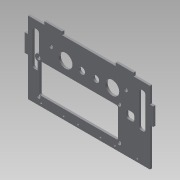
# Autodesk Inventor part: Kepala Tutup belakang
Saved by Autodesk Inventor 2015 SP1 (Build 190203100, 203)
## iProperties
Created: 2015-04-11
Part Number: Kepala Tutup belakang
Material: Generic
Document SubType Name: Modeling
Designer: Rafi Kurnia Putra
Density: 1 g/cm^3
Appearance: Default
Author: Rafi Kurnia Putra
Autodesk Inventor part; units mm, degrees
(part 1 of 2)
ref_plane "YZ Plane" through (0, 0, 0) normal (1, 0, 0) x (0, 1, 0)
ref_plane "XZ Plane" through (0, 0, 0) normal (0, 1, 0) x (-1, 0, 0)
ref_plane "XY Plane" through (0, 0, 0) normal (0, 0, 1) x (1, 0, 0)
sketch "Sketch1" plane through (0, 0, 0) normal (0, 1, 0) x (-1, 0, 0)
  circle A0 centre (-10.5001, 30.1708) radius 1
  circle A1 centre (10.4999, 30.1712) radius 1
  circle A2 centre (23.9063, 30.1714) radius 1
  circle A3 centre (-44.9057, 30.1702) radius 1
  circle A4 centre (44.9063, 30.1718) radius 1
  circle A5 centre (-23.9057, 30.1706) radius 1
  circle A6 centre (47.0718, 65.4919) radius 1.75
  circle A7 centre (47.0718, 34.2919) radius 1.75
  circle A8 centre (-28.1782, 34.2919) radius 1.75
  circle A9 centre (-28.1782, 65.4919) radius 1.75
  circle A10 centre (-6.604, 75.238) radius 3
  circle A11 centre (6.604, 75.238) radius 3
  circle A12 centre (-34.465, 80.373) radius 1.75
  circle A13 centre (35.535, 80.373) radius 1.75
  circle A14 centre (-21.844, 75.746) radius 6.43
  circle A15 centre (21.844, 75.746) radius 6.43
  line L0 (58.58, 79.6254) -> (58.58, 122) construction
  line L1 (-57.0002, 27.1688) -> (-57.0005, 63.0729)
  line L2 (-57.0005, 63.0729) -> (-60.0005, 63.0729)
  line L3 (-60.0005, 63.0729) -> (-60.0005, 79.762)
  line L4 (-60.0005, 79.762) -> (-57.0005, 79.762)
  line L5 (-57.0005, 79.762) -> (-57.0005, 94.8331)
  line L6 (-57.0005, 94.8331) -> (-41.6794, 94.8331)
  line L7 (-41.6794, 94.8331) -> (-41.6794, 97.8331)
  line L8 (-41.6794, 97.8331) -> (-24.9903, 97.8331)
  line L9 (-24.9903, 97.8331) -> (-24.9903, 94.8331)
  line L10 (-24.9903, 94.8331) -> (24.9903, 94.8331)
  line L11 (24.9903, 94.8331) -> (24.9903, 97.8331)
  line L12 (24.9903, 97.8331) -> (41.6794, 97.8331)
  line L13 (41.6794, 97.8331) -> (41.6794, 94.8331)
  line L14 (41.6794, 94.8331) -> (57.0005, 94.8331)
  line L15 (57.0005, 94.8331) -> (57.0005, 79.762)
  line L16 (57.0005, 79.762) -> (59.9995, 79.762)
  line L17 (59.9995, 79.762) -> (59.9998, 63.0742)
  line L18 (59.9998, 63.0742) -> (56.9998, 63.0741)
  line L19 (56.9998, 63.0741) -> (57.0002, 27.1688)
  line L20 (45.2968, 36.8919) -> (-26.4032, 36.8919)
  line L21 (-26.4032, 36.8919) -> (-26.4032, 62.8919)
  line L22 (-26.4032, 62.8919) -> (45.2968, 62.8919)
  line L23 (45.2968, 62.8919) -> (45.2968, 36.8919)
  line L24 (-46.6476, 56.7523) -> (-46.6476, 85.7402)
  line L25 (-48.6476, 87.7402) -> (-50.6476, 87.7402)
  line L26 (-52.6476, 85.7402) -> (-52.6476, 56.7523)
  line L27 (-50.6476, 54.7523) -> (-48.6476, 54.7523)
  arc A16 (-46.6476, 85.7402) -> (-48.6476, 87.7402) centre (-48.6476, 85.7402) ccw
  arc A17 (-50.6476, 87.7402) -> (-52.6476, 85.7402) centre (-50.6476, 85.7402) ccw
  arc A18 (-52.6476, 56.7523) -> (-50.6476, 54.7523) centre (-50.6476, 56.7523) ccw
  arc A19 (-48.6476, 54.7523) -> (-46.6476, 56.7523) centre (-48.6476, 56.7523) ccw
  line L28 (-48.6476, 56.7523) -> (-50.6476, 85.7402) construction
  line L29 (-50.6476, 56.7523) -> (-48.6476, 85.7402) construction
  line L30 (0.035, 14) -> (0.035, 26) construction
  arc A20 (50.7176, 54.7523) -> (52.7176, 56.7523) centre (50.7176, 56.7523) ccw
  arc A21 (46.7176, 56.7523) -> (48.7176, 54.7523) centre (48.7176, 56.7523) ccw
  line L31 (50.7176, 54.7523) -> (48.7176, 54.7523)
  line L32 (52.7176, 85.7402) -> (52.7176, 56.7523)
  arc A22 (48.7176, 87.7402) -> (46.7176, 85.7402) centre (48.7176, 85.7402) ccw
  line L33 (48.7176, 87.7402) -> (50.7176, 87.7402)
  arc A23 (52.7176, 85.7402) -> (50.7176, 87.7402) centre (50.7176, 85.7402) ccw
  line L34 (48.7176, 56.7523) -> (50.7176, 85.7402) construction
  line L35 (50.7176, 56.7523) -> (48.7176, 85.7402) construction
  arc A24 (46.7176, 62.1619) -> (46.7176, 68.822) centre (47.0718, 65.4919) ccw
  line L36 (46.7176, 56.7523) -> (46.7176, 62.1619)
  line L37 (46.7176, 63.7782) -> (46.7176, 62.8919)
  line L38 (46.7176, 68.822) -> (46.7176, 85.7402)
  line L39 (57.0002, 27.1688) -> (-57.0002, 27.1688)
  line L40 (-36.8282, 57.7419) -> (-40.3282, 57.7419)
  line L41 (-42.3282, 59.7419) -> (-42.3282, 63.2419)
  line L42 (-40.3282, 65.2419) -> (-36.8282, 65.2419)
  line L43 (-34.8282, 63.2419) -> (-34.8282, 59.7419)
  line L44 (-34.8282, 57.7419) -> (-42.3282, 65.2419) construction
  line L45 (-42.3282, 57.7419) -> (-34.8282, 65.2419) construction
  arc A25 (-36.8282, 57.7419) -> (-34.8282, 59.7419) centre (-36.8282, 59.7419) ccw
  arc A26 (-42.3282, 59.7419) -> (-40.3282, 57.7419) centre (-40.3282, 59.7419) ccw
  arc A27 (-40.3282, 65.2419) -> (-42.3282, 63.2419) centre (-40.3282, 63.2419) ccw
  arc A28 (-34.8282, 63.2419) -> (-36.8282, 65.2419) centre (-36.8282, 63.2419) ccw
  line L46 (-27.2951, 36) -> (46.1888, 36)
  line L47 (46.1888, 36) -> (46.1888, 63.7839)
  line L48 (46.1888, 63.7839) -> (-27.2951, 63.7839)
  line L49 (-27.2951, 63.7839) -> (-27.2951, 36)
  point P0 (-49.6476, 71.2463)
  point P1 (-60.0005, 71.2463)
  point P2 (49.7176, 71.2463)
  point P3 (0, 73.6476)
  point P4 (-28.274, 68.5919)
  point P5 (35.535, 92.123)
  point P6 (-38.5782, 61.4919)
  dimension "d20" = 6
  dimension "d21" = 0
  dimension "d22" = 7.353
  dimension "d23" = 1.5989
  dimension "d27" = 43.688
  dimension "d28" = 21.844
  dimension "d30" = 3.1
  dimension "d32" = 11.75
  dimension "d33" = 6
  dimension "d34" = 6.604
  dimension "d35" = 6.604
  dimension "d38" = 13.691
  dimension "d45" = 70
  dimension "d52" = 7.5
  dimension "d53" = 2
  dimension "d61" = 26
  dimension "d62" = 71.7
  dimension "d63" = 31.2
  dimension "d64" = 75.25
  dimension "d67" = 2.6
  dimension "d70" = 1.775
  dimension "d71" = 10.4
  dimension "d74" = 0.8919
  constraints: 100 end point, 28 centre point, 26 point on circle, 16 tangent, 13 symmetric about line, 10 point on line, 9 parallel, 4 midpoint, 4 perpendicular, 3 equal radius, 3 horizontal, 2 horizontal alignment, 2 vertical, 2 vertical alignment, 12 other
  measures "d20" distance between parallel lines of L26 L24
  measures "d21" vertical distance of point (-49.648, 71.246) point (-60.001, 71.246)
  measures "d22" distance from line of L1 point (-49.648, 71.246)
  measures "d27" distance of A14.centre A15.centre
  measures "d28" horizontal distance of point (0, 73.648) A15.centre
  measures "d30" vertical distance of point (-28.274, 68.592) A9.centre
  measures "d32" distance of point (35.535, 92.123) A13.centre
  measures "d33" diameter of A10
  measures "d34" horizontal distance of A10.centre point (0, 73.648)
  measures "d35" horizontal distance of A11.centre point (0, 73.648)
  measures "d38" horizontal distance of A15.centre A13.centre
  measures "d45" distance of A12.centre A13.centre
  measures "d52" distance of L45.start L44.end
  measures "d53" radius of A25
  measures "d61" distance between parallel lines of L22 L20
  measures "d62" distance between parallel lines of L21 L23
  measures "d63" distance of A9.centre A8.centre
  measures "d64" distance of A8.centre A7.centre
  measures "d67" distance from line of A7.centre L20
  measures "d70" distance from line of A7.centre L23
  measures "d71" horizontal distance of point (-38.578, 61.492) A9.centre
  measures "d74" distance between parallel lines of L20 L46
extrude "Extrusion1" add sketch "Sketch1" along normal blind 2 contours L1 L2 L3 L4 L5 L6 L7 L8 L9 L10 L11 L12 L13 L14 L15 L16 L17 L18 L19 L39 | L40 A26 L41 A27 L42 A28 L43 A25 | L49 L48 L47 L46
sketch "Sketch2" plane through (0, 2, 0) normal (0, 1, 0) x (1, 0, 0)
  line L0 (-22.4709, -80.6452) -> (21.8526, -80.6452) construction
  line L1 (21.8526, -80.6452) -> (21.8526, -96.7887) construction
  line L2 (21.8526, -96.7887) -> (-22.4709, -96.7887) construction
  line L3 (-22.4709, -96.7887) -> (-22.4709, -80.6452) construction
  line L4 (38.4446, -27.4209) -> (45.2182, -27.4209) construction
  line L5 (45.2182, -27.4209) -> (45.2182, -65.4969) construction
  line L6 (45.2182, -65.4969) -> (38.4446, -65.4969) construction
  line L7 (38.4446, -65.4969) -> (38.4446, -27.4209) construction
  spline S0 degree 2 poles (-35.3902, -91.377) (-36.3991, -91.377) (-37.485, -90.4046) (-37.485, -89.4645) knots 0 0 0 1 2 2 2
  line L8 (-37.485, -89.4645) -> (-37.485, -86.2717)
  line L9 (-37.485, -86.2717) -> (-36.2289, -86.2717)
  line L10 (-36.2289, -86.2717) -> (-36.2289, -89.3916)
  spline S1 degree 2 poles (-36.2289, -89.3916) (-36.2289, -89.9143) (-35.8359, -90.4248) (-35.3902, -90.4248) knots 0 0 0 1 2 2 2
  spline S2 degree 2 poles (-35.3902, -90.4248) (-34.9566, -90.4248) (-34.5514, -89.9346) (-34.5514, -89.3916) knots 0 0 0 1 2 2 2
  line L11 (-34.5514, -89.3916) -> (-34.5514, -86.2717)
  line L12 (-34.5514, -86.2717) -> (-33.2953, -86.2717)
  line L13 (-33.2953, -86.2717) -> (-33.2953, -89.4605)
  spline S3 degree 2 poles (-33.2953, -89.4605) (-33.2953, -90.3843) (-34.3529, -91.377) (-35.3902, -91.377) knots 0 0 0 1 2 2 2
  line L14 (-28.8707, -91.2717) -> (-30.0539, -91.2717)
  line L15 (-30.0539, -91.2717) -> (-30.0539, -89.4038)
  spline S4 degree 2 poles (-30.0539, -89.4038) (-30.0539, -89.1728) (-30.0903, -88.719) (-30.1389, -88.6137) knots 0 0 0 1 2 2 2
  spline S5 degree 2 poles (-30.1389, -88.6137) (-30.1997, -88.484) (-30.4266, -88.3746) (-30.6211, -88.3746) knots 0 0 0 1 2 2 2
  spline S6 degree 2 poles (-30.6211, -88.3746) (-30.7629, -88.3746) (-31.0587, -88.484) (-31.2248, -88.6015) knots 0 0 0 1 2 2 2
  line L16 (-31.2248, -88.6015) -> (-31.2248, -91.2717)
  line L17 (-31.2248, -91.2717) -> (-32.3999, -91.2717)
  line L18 (-32.3999, -91.2717) -> (-32.3999, -87.4994)
  line L19 (-32.3999, -87.4994) -> (-31.2248, -87.4994)
  line L20 (-31.2248, -87.4994) -> (-31.2248, -87.9167)
  spline S7 degree 2 poles (-31.2248, -87.9167) (-30.9372, -87.6736) (-30.3902, -87.3981) (-30.0579, -87.3981) knots 0 0 0 1 2 2 2
  spline S8 degree 2 poles (-30.0579, -87.3981) (-29.4825, -87.3981) (-28.8707, -88.1274) (-28.8707, -88.8162) knots 0 0 0 1 2 2 2
  line L21 (-28.8707, -88.8162) -> (-28.8707, -91.2717)
  line L22 (-26.8245, -91.2717) -> (-27.9996, -91.2717)
  line L23 (-27.9996, -91.2717) -> (-27.9996, -87.4994)
  line L24 (-27.9996, -87.4994) -> (-26.8245, -87.4994)
  line L25 (-26.8245, -87.4994) -> (-26.8245, -91.2717)
  line L26 (-26.788, -86.9605) -> (-28.032, -86.9605)
  line L27 (-28.032, -86.9605) -> (-28.032, -86.0448)
  line L28 (-28.032, -86.0448) -> (-26.788, -86.0448)
  line L29 (-26.788, -86.0448) -> (-26.788, -86.9605)
  line L30 (-22.3958, -87.4994) -> (-23.7492, -91.2717)
  line L31 (-23.7492, -91.2717) -> (-25.0336, -91.2717)
  line L32 (-25.0336, -91.2717) -> (-26.3748, -87.4994)
  line L33 (-26.3748, -87.4994) -> (-25.1389, -87.4994)
  line L34 (-25.1389, -87.4994) -> (-24.3691, -89.9913)
  line L35 (-24.3691, -89.9913) -> (-23.6073, -87.4994)
  line L36 (-23.6073, -87.4994) -> (-22.3958, -87.4994)
  spline S9 degree 2 poles (-20.0133, -91.373) (-21.083, -91.373) (-22.2216, -90.3519) (-22.2216, -89.4078) knots 0 0 0 1 2 2 2
  spline S10 degree 2 poles (-22.2216, -89.4078) (-22.2216, -88.484) (-21.16, -87.3819) (-20.2038, -87.3819) knots 0 0 0 1 2 2 2
  spline S11 degree 2 poles (-20.2038, -87.3819) (-19.3407, -87.3819) (-18.4655, -88.3179) (-18.4655, -89.185) knots 0 0 0 1 2 2 2
  line L37 (-18.4655, -89.185) -> (-18.4655, -89.6104)
  line L38 (-18.4655, -89.6104) -> (-21.0466, -89.6104)
  spline S12 degree 2 poles (-21.0466, -89.6104) (-21.0303, -89.8738) (-20.8399, -90.2222) (-20.6859, -90.3276) knots 0 0 0 1 2 2 2
  spline S13 degree 2 poles (-20.6859, -90.3276) (-20.536, -90.4329) (-20.1308, -90.5221) (-19.8918, -90.5221) knots 0 0 0 1 2 2 2
  spline S14 degree 2 poles (-19.8918, -90.5221) (-19.6892, -90.5221) (-19.2921, -90.4329) (-19.126, -90.356) knots 0 0 0 1 2 2 2
  spline S15 degree 2 poles (-19.126, -90.356) (-18.9801, -90.2952) (-18.737, -90.1453) (-18.66, -90.0885) knots 0 0 0 1 2 2 2
  line L39 (-18.66, -90.0885) -> (-18.5344, -90.0885)
  line L40 (-18.5344, -90.0885) -> (-18.5344, -91.061)
  spline S16 degree 2 poles (-18.5344, -91.061) (-18.6803, -91.1177) (-18.9153, -91.215) (-19.126, -91.2636) knots 0 0 0 1 2 2 2
  spline S17 degree 2 poles (-19.126, -91.2636) (-19.3164, -91.3162) (-19.7216, -91.373) (-20.0133, -91.373) knots 0 0 0 1 2 2 2
  spline S18 degree 2 poles (-19.6244, -88.9013) (-19.6325, -88.5286) (-19.9607, -88.1355) (-20.297, -88.1355) knots 0 0 0 1 2 2 2
  spline S19 degree 2 poles (-20.297, -88.1355) (-20.6414, -88.1355) (-21.0303, -88.5488) (-21.0506, -88.9013) knots 0 0 0 1 2 2 2
  line L41 (-21.0506, -88.9013) -> (-19.6244, -88.9013)
  line L42 (-15.3294, -88.6137) -> (-15.4266, -88.6137)
  spline S20 degree 2 poles (-15.4266, -88.6137) (-15.4955, -88.5893) (-15.7508, -88.565) (-15.9047, -88.565) knots 0 0 0 1 2 2 2
  spline S21 degree 2 poles (-15.9047, -88.565) (-16.0871, -88.565) (-16.4963, -88.6744) (-16.6868, -88.7474) knots 0 0 0 1 2 2 2
  line L43 (-16.6868, -88.7474) -> (-16.6868, -91.2717)
  line L44 (-16.6868, -91.2717) -> (-17.8618, -91.2717)
  line L45 (-17.8618, -91.2717) -> (-17.8618, -87.4994)
  line L46 (-17.8618, -87.4994) -> (-16.6868, -87.4994)
  line L47 (-16.6868, -87.4994) -> (-16.6868, -88.0423)
  spline S22 degree 2 poles (-16.6868, -88.0423) (-16.6057, -87.9694) (-16.3221, -87.7425) (-16.2046, -87.6736) knots 0 0 0 1 2 2 2
  spline S23 degree 2 poles (-16.2046, -87.6736) (-16.0749, -87.5966) (-15.7346, -87.4872) (-15.5846, -87.4872) knots 0 0 0 1 2 2 2
  spline S24 degree 2 poles (-15.5846, -87.4872) (-15.5279, -87.4872) (-15.3861, -87.4953) (-15.3294, -87.4994) knots 0 0 0 1 2 2 2
  line L48 (-15.3294, -87.4994) -> (-15.3294, -88.6137)
  spline S25 degree 2 poles (-13.7329, -91.373) (-14.1462, -91.373) (-14.8877, -91.1906) (-15.1308, -91.0691) knots 0 0 0 1 2 2 2
  line L49 (-15.1308, -91.0691) -> (-15.1308, -90.0764)
  line L50 (-15.1308, -90.0764) -> (-15.0336, -90.0764)
  spline S26 degree 2 poles (-15.0336, -90.0764) (-14.9485, -90.1412) (-14.7338, -90.2952) (-14.5433, -90.3803) knots 0 0 0 1 2 2 2
  spline S27 degree 2 poles (-14.5433, -90.3803) (-14.3772, -90.4573) (-13.968, -90.5667) (-13.7248, -90.5667) knots 0 0 0 1 2 2 2
  spline S28 degree 2 poles (-13.7248, -90.5667) (-13.4777, -90.5667) (-13.0968, -90.4127) (-13.0968, -90.2466) knots 0 0 0 1 2 2 2
  spline S29 degree 2 poles (-13.0968, -90.2466) (-13.0968, -90.1169) (-13.271, -89.9791) (-13.5222, -89.9224) knots 0 0 0 1 2 2 2
  spline S30 degree 2 poles (-13.5222, -89.9224) (-13.656, -89.8859) (-14.0652, -89.809) (-14.2232, -89.7603) knots 0 0 0 1 2 2 2
  spline S31 degree 2 poles (-14.2232, -89.7603) (-14.6689, -89.6226) (-15.1146, -89.0837) (-15.1146, -88.642) knots 0 0 0 1 2 2 2
  spline S32 degree 2 poles (-15.1146, -88.642) (-15.1146, -88.3908) (-14.8837, -87.9451) (-14.6568, -87.7709) knots 0 0 0 1 2 2 2
  spline S33 degree 2 poles (-14.6568, -87.7709) (-14.4339, -87.6007) (-13.7735, -87.3981) (-13.3561, -87.3981) knots 0 0 0 1 2 2 2
  spline S34 degree 2 poles (-13.3561, -87.3981) (-12.959, -87.3981) (-12.2945, -87.5561) (-12.0676, -87.6655) knots 0 0 0 1 2 2 2
  line L51 (-12.0676, -87.6655) -> (-12.0676, -88.6218)
  line L52 (-12.0676, -88.6218) -> (-12.1608, -88.6218)
  spline S35 degree 2 poles (-12.1608, -88.6218) (-12.2216, -88.5731) (-12.485, -88.4151) (-12.6065, -88.3584) knots 0 0 0 1 2 2 2
  spline S36 degree 2 poles (-12.6065, -88.3584) (-12.7564, -88.2936) (-13.1211, -88.2044) (-13.3115, -88.2044) knots 0 0 0 1 2 2 2
  spline S37 degree 2 poles (-13.3115, -88.2044) (-13.5668, -88.2044) (-13.9193, -88.3786) (-13.9193, -88.5205) knots 0 0 0 1 2 2 2
  spline S38 degree 2 poles (-13.9193, -88.5205) (-13.9193, -88.6501) (-13.7451, -88.796) (-13.4534, -88.8689) knots 0 0 0 1 2 2 2
  spline S39 degree 2 poles (-13.4534, -88.8689) (-13.3034, -88.9054) (-12.9104, -88.9743) (-12.7281, -89.035) knots 0 0 0 1 2 2 2
  spline S40 degree 2 poles (-12.7281, -89.035) (-12.3229, -89.1647) (-11.9015, -89.6712) (-11.9015, -90.0926) knots 0 0 0 1 2 2 2
  spline S41 degree 2 poles (-11.9015, -90.0926) (-11.9015, -90.356) (-12.1487, -90.8381) (-12.3796, -91.0002) knots 0 0 0 1 2 2 2
  spline S42 degree 2 poles (-12.3796, -91.0002) (-12.6187, -91.1785) (-13.2751, -91.373) (-13.7329, -91.373) knots 0 0 0 1 2 2 2
  line L53 (-10.1673, -91.2717) -> (-11.3423, -91.2717)
  line L54 (-11.3423, -91.2717) -> (-11.3423, -87.4994)
  line L55 (-11.3423, -87.4994) -> (-10.1673, -87.4994)
  line L56 (-10.1673, -87.4994) -> (-10.1673, -91.2717)
  line L57 (-10.1308, -86.9605) -> (-11.3748, -86.9605)
  line L58 (-11.3748, -86.9605) -> (-11.3748, -86.0448)
  line L59 (-11.3748, -86.0448) -> (-10.1308, -86.0448)
  line L60 (-10.1308, -86.0448) -> (-10.1308, -86.9605)
  spline S43 degree 2 poles (-7.8253, -91.3446) (-8.5425, -91.3446) (-9.1989, -90.753) (-9.1989, -90.0804) knots 0 0 0 1 2 2 2
  line L61 (-9.1989, -90.0804) -> (-9.1989, -88.3179)
  line L62 (-9.1989, -88.3179) -> (-9.6487, -88.3179)
  line L63 (-9.6487, -88.3179) -> (-9.6487, -87.4994)
  line L64 (-9.6487, -87.4994) -> (-9.1989, -87.4994)
  line L65 (-9.1989, -87.4994) -> (-9.1989, -86.4216)
  line L66 (-9.1989, -86.4216) -> (-8.0239, -86.4216)
  line L67 (-8.0239, -86.4216) -> (-8.0239, -87.4994)
  line L68 (-8.0239, -87.4994) -> (-6.8893, -87.4994)
  line L69 (-6.8893, -87.4994) -> (-6.8893, -88.3179)
  line L70 (-6.8893, -88.3179) -> (-8.0239, -88.3179)
  line L71 (-8.0239, -88.3179) -> (-8.0239, -89.659)
  spline S44 degree 2 poles (-8.0239, -89.659) (-8.0239, -89.8576) (-8.0158, -90.1534) (-7.9671, -90.2709) knots 0 0 0 1 2 2 2
  spline S45 degree 2 poles (-7.9671, -90.2709) (-7.9185, -90.3884) (-7.6795, -90.5261) (-7.4526, -90.5261) knots 0 0 0 1 2 2 2
  spline S46 degree 2 poles (-7.4526, -90.5261) (-7.3553, -90.5261) (-7.0514, -90.4451) (-6.9906, -90.4127) knots 0 0 0 1 2 2 2
  line L72 (-6.9906, -90.4127) -> (-6.8893, -90.4127)
  line L73 (-6.8893, -90.4127) -> (-6.8893, -91.2393)
  spline S47 degree 2 poles (-6.8893, -91.2393) (-7.0798, -91.2879) (-7.5093, -91.3446) (-7.8253, -91.3446) knots 0 0 0 1 2 2 2
  spline S48 degree 2 poles (-4.3326, -90.8705) (-4.4542, -90.9718) (-4.6446, -91.1339) (-4.8067, -91.215) knots 0 0 0 1 2 2 2
  spline S49 degree 2 poles (-4.8067, -91.215) (-4.9647, -91.2919) (-5.2645, -91.373) (-5.532, -91.373) knots 0 0 0 1 2 2 2
  spline S50 degree 2 poles (-5.532, -91.373) (-6.0344, -91.373) (-6.6949, -90.7004) (-6.6949, -90.1898) knots 0 0 0 1 2 2 2
  spline S51 degree 2 poles (-6.6949, -90.1898) (-6.6949, -89.7725) (-6.3586, -89.2538) (-6.0425, -89.1039) knots 0 0 0 1 2 2 2
  spline S52 degree 2 poles (-6.0425, -89.1039) (-5.7224, -88.95) (-4.8351, -88.8284) (-4.3245, -88.796) knots 0 0 0 1 2 2 2
  line L74 (-4.3245, -88.796) -> (-4.3245, -88.7757)
  spline S53 degree 2 poles (-4.3245, -88.7757) (-4.3245, -88.4637) (-4.7864, -88.2247) (-5.2483, -88.2247) knots 0 0 0 1 2 2 2
  spline S54 degree 2 poles (-5.2483, -88.2247) (-5.455, -88.2247) (-6.0141, -88.3746) (-6.2775, -88.4921) knots 0 0 0 1 2 2 2
  line L75 (-6.2775, -88.4921) -> (-6.3788, -88.4921)
  line L76 (-6.3788, -88.4921) -> (-6.3788, -87.5804)
  spline S55 degree 2 poles (-6.3788, -87.5804) (-6.2046, -87.5318) (-5.4266, -87.394) (-5.0295, -87.394) knots 0 0 0 1 2 2 2
  spline S56 degree 2 poles (-5.0295, -87.394) (-4.0571, -87.394) (-3.1657, -88.0423) (-3.1657, -88.7068) knots 0 0 0 1 2 2 2
  line L77 (-3.1657, -88.7068) -> (-3.1657, -91.2717)
  line L78 (-3.1657, -91.2717) -> (-4.3326, -91.2717)
  line L79 (-4.3326, -91.2717) -> (-4.3326, -90.8705)
  line L80 (-4.3326, -90.2871) -> (-4.3326, -89.5051)
  spline S57 degree 2 poles (-4.3326, -89.5051) (-4.6325, -89.5334) (-5.0012, -89.578) (-5.1795, -89.6428) knots 0 0 0 1 2 2 2
  spline S58 degree 2 poles (-5.1795, -89.6428) (-5.3375, -89.6955) (-5.5077, -89.9143) (-5.5077, -90.0926) knots 0 0 0 1 2 2 2
  spline S59 degree 2 poles (-5.5077, -90.0926) (-5.5077, -90.356) (-5.22, -90.5545) (-4.9404, -90.5545) knots 0 0 0 1 2 2 2
  spline S60 degree 2 poles (-4.9404, -90.5545) (-4.7864, -90.5545) (-4.4623, -90.4127) (-4.3326, -90.2871) knots 0 0 0 1 2 2 2
  spline S61 degree 2 poles (-1.1479, -91.373) (-1.5611, -91.373) (-2.3026, -91.1906) (-2.5457, -91.0691) knots 0 0 0 1 2 2 2
  line L81 (-2.5457, -91.0691) -> (-2.5457, -90.0764)
  line L82 (-2.5457, -90.0764) -> (-2.4485, -90.0764)
  spline S62 degree 2 poles (-2.4485, -90.0764) (-2.3634, -90.1412) (-2.1487, -90.2952) (-1.9582, -90.3803) knots 0 0 0 1 2 2 2
  spline S63 degree 2 poles (-1.9582, -90.3803) (-1.7921, -90.4573) (-1.3829, -90.5667) (-1.1398, -90.5667) knots 0 0 0 1 2 2 2
  spline S64 degree 2 poles (-1.1398, -90.5667) (-0.8926, -90.5667) (-0.5117, -90.4127) (-0.5117, -90.2466) knots 0 0 0 1 2 2 2
  spline S65 degree 2 poles (-0.5117, -90.2466) (-0.5117, -90.1169) (-0.6859, -89.9791) (-0.9372, -89.9224) knots 0 0 0 1 2 2 2
  spline S66 degree 2 poles (-0.9372, -89.9224) (-1.0709, -89.8859) (-1.4801, -89.809) (-1.6381, -89.7603) knots 0 0 0 1 2 2 2
  spline S67 degree 2 poles (-1.6381, -89.7603) (-2.0838, -89.6226) (-2.5295, -89.0837) (-2.5295, -88.642) knots 0 0 0 1 2 2 2
  spline S68 degree 2 poles (-2.5295, -88.642) (-2.5295, -88.3908) (-2.2986, -87.9451) (-2.0717, -87.7709) knots 0 0 0 1 2 2 2
  spline S69 degree 2 poles (-2.0717, -87.7709) (-1.8488, -87.6007) (-1.1884, -87.3981) (-0.771, -87.3981) knots 0 0 0 1 2 2 2
  spline S70 degree 2 poles (-0.771, -87.3981) (-0.3739, -87.3981) (0.2906, -87.5561) (0.5175, -87.6655) knots 0 0 0 1 2 2 2
  line L83 (0.5175, -87.6655) -> (0.5175, -88.6218)
  line L84 (0.5175, -88.6218) -> (0.4243, -88.6218)
  spline S71 degree 2 poles (0.4243, -88.6218) (0.3635, -88.5731) (0.1001, -88.4151) (-0.0214, -88.3584) knots 0 0 0 1 2 2 2
  spline S72 degree 2 poles (-0.0214, -88.3584) (-0.1714, -88.2936) (-0.536, -88.2044) (-0.7265, -88.2044) knots 0 0 0 1 2 2 2
  spline S73 degree 2 poles (-0.7265, -88.2044) (-0.9817, -88.2044) (-1.3342, -88.3786) (-1.3342, -88.5205) knots 0 0 0 1 2 2 2
  spline S74 degree 2 poles (-1.3342, -88.5205) (-1.3342, -88.6501) (-1.16, -88.796) (-0.8683, -88.8689) knots 0 0 0 1 2 2 2
  spline S75 degree 2 poles (-0.8683, -88.8689) (-0.7184, -88.9054) (-0.3253, -88.9743) (-0.143, -89.035) knots 0 0 0 1 2 2 2
  spline S76 degree 2 poles (-0.143, -89.035) (0.2622, -89.1647) (0.6836, -89.6712) (0.6836, -90.0926) knots 0 0 0 1 2 2 2
  spline S77 degree 2 poles (0.6836, -90.0926) (0.6836, -90.356) (0.4364, -90.8381) (0.2055, -91.0002) knots 0 0 0 1 2 2 2
  spline S78 degree 2 poles (0.2055, -91.0002) (-0.0336, -91.1785) (-0.69, -91.373) (-1.1479, -91.373) knots 0 0 0 1 2 2 2
  line L85 (5.8132, -91.2717) -> (3.1228, -91.2717)
  line L86 (3.1228, -91.2717) -> (3.1228, -90.4005)
  line L87 (3.1228, -90.4005) -> (3.84, -90.4005)
  line L88 (3.84, -90.4005) -> (3.84, -87.1428)
  line L89 (3.84, -87.1428) -> (3.1228, -87.1428)
  line L90 (3.1228, -87.1428) -> (3.1228, -86.2717)
  line L91 (3.1228, -86.2717) -> (5.8132, -86.2717)
  line L92 (5.8132, -86.2717) -> (5.8132, -87.1428)
  line L93 (5.8132, -87.1428) -> (5.0961, -87.1428)
  line L94 (5.0961, -87.1428) -> (5.0961, -90.4005)
  line L95 (5.0961, -90.4005) -> (5.8132, -90.4005)
  line L96 (5.8132, -90.4005) -> (5.8132, -91.2717)
  line L97 (10.1082, -91.2717) -> (8.9251, -91.2717)
  line L98 (8.9251, -91.2717) -> (8.9251, -89.4038)
  spline S79 degree 2 poles (8.9251, -89.4038) (8.9251, -89.1728) (8.8886, -88.719) (8.84, -88.6137) knots 0 0 0 1 2 2 2
  spline S80 degree 2 poles (8.84, -88.6137) (8.7792, -88.484) (8.5523, -88.3746) (8.3578, -88.3746) knots 0 0 0 1 2 2 2
  spline S81 degree 2 poles (8.3578, -88.3746) (8.216, -88.3746) (7.9202, -88.484) (7.7541, -88.6015) knots 0 0 0 1 2 2 2
  line L99 (7.7541, -88.6015) -> (7.7541, -91.2717)
  line L100 (7.7541, -91.2717) -> (6.5791, -91.2717)
  line L101 (6.5791, -91.2717) -> (6.5791, -87.4994)
  line L102 (6.5791, -87.4994) -> (7.7541, -87.4994)
  line L103 (7.7541, -87.4994) -> (7.7541, -87.9167)
  spline S82 degree 2 poles (7.7541, -87.9167) (8.0418, -87.6736) (8.5888, -87.3981) (8.921, -87.3981) knots 0 0 0 1 2 2 2
  spline S83 degree 2 poles (8.921, -87.3981) (9.4964, -87.3981) (10.1082, -88.1274) (10.1082, -88.8162) knots 0 0 0 1 2 2 2
  line L104 (10.1082, -88.8162) -> (10.1082, -91.2717)
  line L105 (14.4073, -91.2717) -> (13.2322, -91.2717)
  line L106 (13.2322, -91.2717) -> (13.2322, -90.8786)
  spline S84 degree 2 poles (13.2322, -90.8786) (13.1188, -90.9718) (12.827, -91.1866) (12.7136, -91.2433) knots 0 0 0 1 2 2 2
  spline S85 degree 2 poles (12.7136, -91.2433) (12.5758, -91.3081) (12.3003, -91.377) (12.1098, -91.377) knots 0 0 0 1 2 2 2
  spline S86 degree 2 poles (12.1098, -91.377) (11.4656, -91.377) (10.712, -90.3073) (10.712, -89.4159) knots 0 0 0 1 2 2 2
  spline S87 degree 2 poles (10.712, -89.4159) (10.712, -88.9216) (10.9672, -88.1963) (11.1901, -87.9289) knots 0 0 0 1 2 2 2
  spline S88 degree 2 poles (11.1901, -87.9289) (11.3967, -87.6817) (11.9802, -87.3981) (12.3043, -87.3981) knots 0 0 0 1 2 2 2
  spline S89 degree 2 poles (12.3043, -87.3981) (12.6001, -87.3981) (12.981, -87.5237) (13.2322, -87.6534) knots 0 0 0 1 2 2 2
  line L107 (13.2322, -87.6534) -> (13.2322, -86.0488)
  line L108 (13.2322, -86.0488) -> (14.4073, -86.0488)
  line L109 (14.4073, -86.0488) -> (14.4073, -91.2717)
  line L110 (13.2322, -90.2344) -> (13.2322, -88.3827)
  spline S90 degree 2 poles (13.2322, -88.3827) (13.1471, -88.3381) (12.8635, -88.2814) (12.7622, -88.2814) knots 0 0 0 1 2 2 2
  spline S91 degree 2 poles (12.7622, -88.2814) (12.3408, -88.2814) (11.9154, -88.873) (11.9154, -89.4038) knots 0 0 0 1 2 2 2
  spline S92 degree 2 poles (11.9154, -89.4038) (11.9154, -89.9629) (12.2557, -90.4613) (12.6325, -90.4613) knots 0 0 0 1 2 2 2
  spline S93 degree 2 poles (12.6325, -90.4613) (12.7865, -90.4613) (13.1026, -90.3397) (13.2322, -90.2344) knots 0 0 0 1 2 2 2
  spline S94 degree 2 poles (18.9251, -89.3876) (18.9251, -90.3195) (17.9081, -91.3892) (16.9802, -91.3892) knots 0 0 0 1 2 2 2
  spline S95 degree 2 poles (16.9802, -91.3892) (16.0564, -91.3892) (15.0312, -90.3195) (15.0312, -89.3876) knots 0 0 0 1 2 2 2
  spline S96 degree 2 poles (15.0312, -89.3876) (15.0312, -88.4475) (16.0564, -87.3819) (16.9802, -87.3819) knots 0 0 0 1 2 2 2
  spline S97 degree 2 poles (16.9802, -87.3819) (17.904, -87.3819) (18.9251, -88.4516) (18.9251, -89.3876) knots 0 0 0 1 2 2 2
  spline S98 degree 2 poles (17.7217, -89.3957) (17.7217, -89.0594) (17.6123, -88.6096) (17.515, -88.4759) knots 0 0 0 1 2 2 2
  spline S99 degree 2 poles (17.515, -88.4759) (17.4097, -88.3341) (17.1463, -88.2247) (16.9802, -88.2247) knots 0 0 0 1 2 2 2
  spline S100 degree 2 poles (16.9802, -88.2247) (16.8181, -88.2247) (16.5628, -88.3219) (16.4575, -88.4597) knots 0 0 0 1 2 2 2
  spline S101 degree 2 poles (16.4575, -88.4597) (16.3562, -88.5893) (16.2346, -89.0472) (16.2346, -89.3957) knots 0 0 0 1 2 2 2
  spline S102 degree 2 poles (16.2346, -89.3957) (16.2346, -89.7401) (16.3481, -90.1655) (16.4413, -90.2952) knots 0 0 0 1 2 2 2
  spline S103 degree 2 poles (16.4413, -90.2952) (16.5345, -90.4248) (16.8181, -90.5464) (16.9883, -90.5464) knots 0 0 0 1 2 2 2
  spline S104 degree 2 poles (16.9883, -90.5464) (17.1301, -90.5464) (17.4218, -90.4248) (17.511, -90.3033) knots 0 0 0 1 2 2 2
  spline S105 degree 2 poles (17.511, -90.3033) (17.6123, -90.1615) (17.7217, -89.7522) (17.7217, -89.3957) knots 0 0 0 1 2 2 2
  line L111 (23.0782, -91.2717) -> (21.8951, -91.2717)
  line L112 (21.8951, -91.2717) -> (21.8951, -89.4038)
  spline S106 degree 2 poles (21.8951, -89.4038) (21.8951, -89.1728) (21.8586, -88.719) (21.81, -88.6137) knots 0 0 0 1 2 2 2
  spline S107 degree 2 poles (21.81, -88.6137) (21.7492, -88.484) (21.5223, -88.3746) (21.3278, -88.3746) knots 0 0 0 1 2 2 2
  spline S108 degree 2 poles (21.3278, -88.3746) (21.186, -88.3746) (20.8902, -88.484) (20.7241, -88.6015) knots 0 0 0 1 2 2 2
  line L113 (20.7241, -88.6015) -> (20.7241, -91.2717)
  line L114 (20.7241, -91.2717) -> (19.5491, -91.2717)
  line L115 (19.5491, -91.2717) -> (19.5491, -87.4994)
  line L116 (19.5491, -87.4994) -> (20.7241, -87.4994)
  line L117 (20.7241, -87.4994) -> (20.7241, -87.9167)
  spline S109 degree 2 poles (20.7241, -87.9167) (21.0118, -87.6736) (21.5588, -87.3981) (21.891, -87.3981) knots 0 0 0 1 2 2 2
  spline S110 degree 2 poles (21.891, -87.3981) (22.4664, -87.3981) (23.0782, -88.1274) (23.0782, -88.8162) knots 0 0 0 1 2 2 2
  line L118 (23.0782, -88.8162) -> (23.0782, -91.2717)
  spline S111 degree 2 poles (25.8821, -91.373) (24.8124, -91.373) (23.6739, -90.3519) (23.6739, -89.4078) knots 0 0 0 1 2 2 2
  spline S112 degree 2 poles (23.6739, -89.4078) (23.6739, -88.484) (24.7355, -87.3819) (25.6917, -87.3819) knots 0 0 0 1 2 2 2
  spline S113 degree 2 poles (25.6917, -87.3819) (26.5547, -87.3819) (27.4299, -88.3179) (27.4299, -89.185) knots 0 0 0 1 2 2 2
  line L119 (27.4299, -89.185) -> (27.4299, -89.6104)
  line L120 (27.4299, -89.6104) -> (24.8489, -89.6104)
  spline S114 degree 2 poles (24.8489, -89.6104) (24.8651, -89.8738) (25.0555, -90.2222) (25.2095, -90.3276) knots 0 0 0 1 2 2 2
  spline S115 degree 2 poles (25.2095, -90.3276) (25.3594, -90.4329) (25.7646, -90.5221) (26.0037, -90.5221) knots 0 0 0 1 2 2 2
  spline S116 degree 2 poles (26.0037, -90.5221) (26.2063, -90.5221) (26.6034, -90.4329) (26.7695, -90.356) knots 0 0 0 1 2 2 2
  spline S117 degree 2 poles (26.7695, -90.356) (26.9154, -90.2952) (27.1585, -90.1453) (27.2355, -90.0885) knots 0 0 0 1 2 2 2
  line L121 (27.2355, -90.0885) -> (27.3611, -90.0885)
  line L122 (27.3611, -90.0885) -> (27.3611, -91.061)
  spline S118 degree 2 poles (27.3611, -91.061) (27.2152, -91.1177) (26.9802, -91.215) (26.7695, -91.2636) knots 0 0 0 1 2 2 2
  spline S119 degree 2 poles (26.7695, -91.2636) (26.5791, -91.3162) (26.1739, -91.373) (25.8821, -91.373) knots 0 0 0 1 2 2 2
  spline S120 degree 2 poles (26.2711, -88.9013) (26.263, -88.5286) (25.9348, -88.1355) (25.5985, -88.1355) knots 0 0 0 1 2 2 2
  spline S121 degree 2 poles (25.5985, -88.1355) (25.2541, -88.1355) (24.8651, -88.5488) (24.8449, -88.9013) knots 0 0 0 1 2 2 2
  line L123 (24.8449, -88.9013) -> (26.2711, -88.9013)
  spline S122 degree 2 poles (29.1803, -91.373) (28.7671, -91.373) (28.0256, -91.1906) (27.7825, -91.0691) knots 0 0 0 1 2 2 2
  line L124 (27.7825, -91.0691) -> (27.7825, -90.0764)
  line L125 (27.7825, -90.0764) -> (27.8797, -90.0764)
  spline S123 degree 2 poles (27.8797, -90.0764) (27.9648, -90.1412) (28.1795, -90.2952) (28.37, -90.3803) knots 0 0 0 1 2 2 2
  spline S124 degree 2 poles (28.37, -90.3803) (28.5361, -90.4573) (28.9453, -90.5667) (29.1885, -90.5667) knots 0 0 0 1 2 2 2
  spline S125 degree 2 poles (29.1885, -90.5667) (29.4356, -90.5667) (29.8165, -90.4127) (29.8165, -90.2466) knots 0 0 0 1 2 2 2
  spline S126 degree 2 poles (29.8165, -90.2466) (29.8165, -90.1169) (29.6423, -89.9791) (29.391, -89.9224) knots 0 0 0 1 2 2 2
  spline S127 degree 2 poles (29.391, -89.9224) (29.2573, -89.8859) (28.8481, -89.809) (28.6901, -89.7603) knots 0 0 0 1 2 2 2
  spline S128 degree 2 poles (28.6901, -89.7603) (28.2444, -89.6226) (27.7987, -89.0837) (27.7987, -88.642) knots 0 0 0 1 2 2 2
  spline S129 degree 2 poles (27.7987, -88.642) (27.7987, -88.3908) (28.0296, -87.9451) (28.2565, -87.7709) knots 0 0 0 1 2 2 2
  spline S130 degree 2 poles (28.2565, -87.7709) (28.4794, -87.6007) (29.1398, -87.3981) (29.5572, -87.3981) knots 0 0 0 1 2 2 2
  spline S131 degree 2 poles (29.5572, -87.3981) (29.9543, -87.3981) (30.6188, -87.5561) (30.8457, -87.6655) knots 0 0 0 1 2 2 2
  line L126 (30.8457, -87.6655) -> (30.8457, -88.6218)
  line L127 (30.8457, -88.6218) -> (30.7525, -88.6218)
  spline S132 degree 2 poles (30.7525, -88.6218) (30.6917, -88.5731) (30.4283, -88.4151) (30.3068, -88.3584) knots 0 0 0 1 2 2 2
  spline S133 degree 2 poles (30.3068, -88.3584) (30.1568, -88.2936) (29.7922, -88.2044) (29.6017, -88.2044) knots 0 0 0 1 2 2 2
  spline S134 degree 2 poles (29.6017, -88.2044) (29.3465, -88.2044) (28.994, -88.3786) (28.994, -88.5205) knots 0 0 0 1 2 2 2
  spline S135 degree 2 poles (28.994, -88.5205) (28.994, -88.6501) (29.1682, -88.796) (29.4599, -88.8689) knots 0 0 0 1 2 2 2
  spline S136 degree 2 poles (29.4599, -88.8689) (29.6098, -88.9054) (30.0029, -88.9743) (30.1852, -89.035) knots 0 0 0 1 2 2 2
  spline S137 degree 2 poles (30.1852, -89.035) (30.5904, -89.1647) (31.0118, -89.6712) (31.0118, -90.0926) knots 0 0 0 1 2 2 2
  spline S138 degree 2 poles (31.0118, -90.0926) (31.0118, -90.356) (30.7646, -90.8381) (30.5337, -91.0002) knots 0 0 0 1 2 2 2
  spline S139 degree 2 poles (30.5337, -91.0002) (30.2946, -91.1785) (29.6382, -91.373) (29.1803, -91.373) knots 0 0 0 1 2 2 2
  line L128 (32.746, -91.2717) -> (31.5709, -91.2717)
  line L129 (31.5709, -91.2717) -> (31.5709, -87.4994)
  line L130 (31.5709, -87.4994) -> (32.746, -87.4994)
  line L131 (32.746, -87.4994) -> (32.746, -91.2717)
  line L132 (32.7825, -86.9605) -> (31.5385, -86.9605)
  line L133 (31.5385, -86.9605) -> (31.5385, -86.0448)
  line L134 (31.5385, -86.0448) -> (32.7825, -86.0448)
  line L135 (32.7825, -86.0448) -> (32.7825, -86.9605)
  spline S140 degree 2 poles (35.7241, -90.8705) (35.6026, -90.9718) (35.4121, -91.1339) (35.25, -91.215) knots 0 0 0 1 2 2 2
  spline S141 degree 2 poles (35.25, -91.215) (35.092, -91.2919) (34.7922, -91.373) (34.5248, -91.373) knots 0 0 0 1 2 2 2
  spline S142 degree 2 poles (34.5248, -91.373) (34.0223, -91.373) (33.3619, -90.7004) (33.3619, -90.1898) knots 0 0 0 1 2 2 2
  spline S143 degree 2 poles (33.3619, -90.1898) (33.3619, -89.7725) (33.6982, -89.2538) (34.0142, -89.1039) knots 0 0 0 1 2 2 2
  spline S144 degree 2 poles (34.0142, -89.1039) (34.3343, -88.95) (35.2217, -88.8284) (35.7322, -88.796) knots 0 0 0 1 2 2 2
  line L136 (35.7322, -88.796) -> (35.7322, -88.7757)
  spline S145 degree 2 poles (35.7322, -88.7757) (35.7322, -88.4637) (35.2703, -88.2247) (34.8084, -88.2247) knots 0 0 0 1 2 2 2
  spline S146 degree 2 poles (34.8084, -88.2247) (34.6017, -88.2247) (34.0426, -88.3746) (33.7792, -88.4921) knots 0 0 0 1 2 2 2
  line L137 (33.7792, -88.4921) -> (33.6779, -88.4921)
  line L138 (33.6779, -88.4921) -> (33.6779, -87.5804)
  spline S147 degree 2 poles (33.6779, -87.5804) (33.8521, -87.5318) (34.6301, -87.394) (35.0272, -87.394) knots 0 0 0 1 2 2 2
  spline S148 degree 2 poles (35.0272, -87.394) (35.9996, -87.394) (36.891, -88.0423) (36.891, -88.7068) knots 0 0 0 1 2 2 2
  line L139 (36.891, -88.7068) -> (36.891, -91.2717)
  line L140 (36.891, -91.2717) -> (35.7241, -91.2717)
  line L141 (35.7241, -91.2717) -> (35.7241, -90.8705)
  line L142 (35.7241, -90.2871) -> (35.7241, -89.5051)
  spline S149 degree 2 poles (35.7241, -89.5051) (35.4243, -89.5334) (35.0555, -89.578) (34.8773, -89.6428) knots 0 0 0 1 2 2 2
  spline S150 degree 2 poles (34.8773, -89.6428) (34.7192, -89.6955) (34.5491, -89.9143) (34.5491, -90.0926) knots 0 0 0 1 2 2 2
  spline S151 degree 2 poles (34.5491, -90.0926) (34.5491, -90.356) (34.8367, -90.5545) (35.1163, -90.5545) knots 0 0 0 1 2 2 2
  spline S152 degree 2 poles (35.1163, -90.5545) (35.2703, -90.5545) (35.5944, -90.4127) (35.7241, -90.2871) knots 0 0 0 1 2 2 2
  line L143 (33.738, -48.2089) -> (32.6687, -48.2089)
  line L144 (32.6687, -48.2089) -> (31.6959, -46.924)
  line L145 (31.6959, -46.924) -> (31.3782, -46.924)
  line L146 (31.3782, -46.924) -> (31.3782, -48.2089)
  line L147 (31.3782, -48.2089) -> (30.5046, -48.2089)
  line L148 (30.5046, -48.2089) -> (30.5046, -44.7089)
  line L149 (30.5046, -44.7089) -> (31.9114, -44.7089)
  spline S153 degree 2 poles (31.9114, -44.7089) (32.2036, -44.7089) (32.6347, -44.7826) (32.819, -44.8961) knots 0 0 0 1 2 2 2
  spline S154 degree 2 poles (32.819, -44.8961) (33.0062, -45.0152) (33.2275, -45.3868) (33.2275, -45.6704) knots 0 0 0 1 2 2 2
  spline S155 degree 2 poles (33.2275, -45.6704) (33.2275, -46.0703) (32.8644, -46.5723) (32.5609, -46.7198) knots 0 0 0 1 2 2 2
  line L150 (32.5609, -46.7198) -> (33.738, -48.2089)
  spline S156 degree 2 poles (32.3255, -45.781) (32.3255, -45.6477) (32.2234, -45.4577) (32.1071, -45.4066) knots 0 0 0 1 2 2 2
  spline S157 degree 2 poles (32.1071, -45.4066) (32.0249, -45.3726) (31.8235, -45.3527) (31.6732, -45.3527) knots 0 0 0 1 2 2 2
  line L151 (31.6732, -45.3527) -> (31.3782, -45.3527)
  line L152 (31.3782, -45.3527) -> (31.3782, -46.2944)
  line L153 (31.3782, -46.2944) -> (31.6306, -46.2944)
  spline S158 degree 2 poles (31.6306, -46.2944) (31.8121, -46.2944) (32.0702, -46.249) (32.1582, -46.1781) knots 0 0 0 1 2 2 2
  spline S159 degree 2 poles (32.1582, -46.1781) (32.2433, -46.11) (32.3255, -45.9285) (32.3255, -45.781) knots 0 0 0 1 2 2 2
  spline S160 degree 2 poles (37.1841, -46.4589) (37.1841, -47.3098) (36.2765, -48.2826) (35.488, -48.2826) knots 0 0 0 1 2 2 2
  spline S161 degree 2 poles (35.488, -48.2826) (34.6967, -48.2826) (33.7947, -47.2984) (33.7947, -46.4589) knots 0 0 0 1 2 2 2
  spline S162 degree 2 poles (33.7947, -46.4589) (33.7947, -45.6165) (34.6967, -44.6351) (35.488, -44.6351) knots 0 0 0 1 2 2 2
  spline S163 degree 2 poles (35.488, -44.6351) (36.2765, -44.6351) (37.1841, -45.6108) (37.1841, -46.4589) knots 0 0 0 1 2 2 2
  spline S164 degree 2 poles (36.2765, -46.4589) (36.2765, -46.1441) (36.1489, -45.7044) (36.0382, -45.5654) knots 0 0 0 1 2 2 2
  spline S165 degree 2 poles (36.0382, -45.5654) (35.9276, -45.4208) (35.644, -45.296) (35.4908, -45.296) knots 0 0 0 1 2 2 2
  spline S166 degree 2 poles (35.4908, -45.296) (35.3292, -45.296) (35.0654, -45.4123) (34.9434, -45.5598) knots 0 0 0 1 2 2 2
  spline S167 degree 2 poles (34.9434, -45.5598) (34.8356, -45.6959) (34.7023, -46.1469) (34.7023, -46.4589) knots 0 0 0 1 2 2 2
  spline S168 degree 2 poles (34.7023, -46.4589) (34.7023, -46.7822) (34.83, -47.2077) (34.9406, -47.3523) knots 0 0 0 1 2 2 2
  spline S169 degree 2 poles (34.9406, -47.3523) (35.0512, -47.497) (35.3377, -47.6218) (35.4908, -47.6218) knots 0 0 0 1 2 2 2
  spline S170 degree 2 poles (35.4908, -47.6218) (35.6468, -47.6218) (35.9361, -47.4885) (36.0411, -47.3466) knots 0 0 0 1 2 2 2
  spline S171 degree 2 poles (36.0411, -47.3466) (36.1545, -47.1935) (36.2765, -46.7879) (36.2765, -46.4589) knots 0 0 0 1 2 2 2
  spline S172 degree 2 poles (40.5026, -47.1368) (40.5026, -47.3977) (40.304, -47.7919) (40.1395, -47.9224) knots 0 0 0 1 2 2 2
  spline S173 degree 2 poles (40.1395, -47.9224) (39.941, -48.0784) (39.4702, -48.2089) (39.1043, -48.2089) knots 0 0 0 1 2 2 2
  line L154 (39.1043, -48.2089) -> (37.706, -48.2089)
  line L155 (37.706, -48.2089) -> (37.706, -44.7089)
  line L156 (37.706, -44.7089) -> (38.9398, -44.7089)
  spline S174 degree 2 poles (38.9398, -44.7089) (39.3255, -44.7089) (39.7226, -44.7684) (39.8956, -44.862) knots 0 0 0 1 2 2 2
  spline S175 degree 2 poles (39.8956, -44.862) (40.0856, -44.9613) (40.27, -45.3017) (40.27, -45.5229) knots 0 0 0 1 2 2 2
  spline S176 degree 2 poles (40.27, -45.5229) (40.27, -45.7782) (40.0147, -46.1781) (39.7878, -46.2717) knots 0 0 0 1 2 2 2
  line L157 (39.7878, -46.2717) -> (39.7878, -46.2887)
  spline S177 degree 2 poles (39.7878, -46.2887) (40.114, -46.3568) (40.5026, -46.7794) (40.5026, -47.1368) knots 0 0 0 1 2 2 2
  spline S178 degree 2 poles (39.595, -47.1226) (39.595, -46.9581) (39.4645, -46.7737) (39.334, -46.7255) knots 0 0 0 1 2 2 2
  spline S179 degree 2 poles (39.334, -46.7255) (39.2546, -46.6943) (38.9738, -46.6886) (38.7412, -46.6886) knots 0 0 0 1 2 2 2
  line L158 (38.7412, -46.6886) -> (38.5796, -46.6886)
  line L159 (38.5796, -46.6886) -> (38.5796, -47.5707)
  line L160 (38.5796, -47.5707) -> (38.6278, -47.5707)
  spline S180 degree 2 poles (38.6278, -47.5707) (38.9681, -47.5707) (39.2291, -47.5622) (39.3652, -47.5026) knots 0 0 0 1 2 2 2
  spline S181 degree 2 poles (39.3652, -47.5026) (39.4843, -47.4488) (39.595, -47.2502) (39.595, -47.1226) knots 0 0 0 1 2 2 2
  spline S182 degree 2 poles (39.3766, -45.6959) (39.3766, -45.6108) (39.2886, -45.4321) (39.1979, -45.3924) knots 0 0 0 1 2 2 2
  spline S183 degree 2 poles (39.1979, -45.3924) (39.1128, -45.3527) (38.8745, -45.3471) (38.6391, -45.3471) knots 0 0 0 1 2 2 2
  line L161 (38.6391, -45.3471) -> (38.5796, -45.3471)
  line L162 (38.5796, -45.3471) -> (38.5796, -46.0902)
  line L163 (38.5796, -46.0902) -> (38.6902, -46.0902)
  spline S184 degree 2 poles (38.6902, -46.0902) (38.9143, -46.0902) (39.0958, -46.0817) (39.1922, -46.0363) knots 0 0 0 1 2 2 2
  spline S185 degree 2 poles (39.1922, -46.0363) (39.2972, -45.9852) (39.3766, -45.8122) (39.3766, -45.6959) knots 0 0 0 1 2 2 2
  spline S186 degree 2 poles (42.4228, -48.2826) (41.7165, -48.2826) (40.9564, -47.6019) (40.9564, -46.9439) knots 0 0 0 1 2 2 2
  line L164 (40.9564, -46.9439) -> (40.9564, -44.7089)
  line L165 (40.9564, -44.7089) -> (41.8356, -44.7089)
  line L166 (41.8356, -44.7089) -> (41.8356, -46.8928)
  spline S187 degree 2 poles (41.8356, -46.8928) (41.8356, -47.2587) (42.1108, -47.6161) (42.4228, -47.6161) knots 0 0 0 1 2 2 2
  spline S188 degree 2 poles (42.4228, -47.6161) (42.7262, -47.6161) (43.0099, -47.2729) (43.0099, -46.8928) knots 0 0 0 1 2 2 2
  line L167 (43.0099, -46.8928) -> (43.0099, -44.7089)
  line L168 (43.0099, -44.7089) -> (43.8891, -44.7089)
  line L169 (43.8891, -44.7089) -> (43.8891, -46.9411)
  spline S189 degree 2 poles (43.8891, -46.9411) (43.8891, -47.5877) (43.1489, -48.2826) (42.4228, -48.2826) knots 0 0 0 1 2 2 2
  spline S190 degree 2 poles (45.6448, -48.2713) (45.242, -48.2713) (44.6351, -48.1153) (44.3741, -48.0018) knots 0 0 0 1 2 2 2
  line L170 (44.3741, -48.0018) -> (44.3741, -47.168)
  line L171 (44.3741, -47.168) -> (44.4536, -47.168)
  spline S191 degree 2 poles (44.4536, -47.168) (44.7173, -47.392) (45.3498, -47.6331) (45.6476, -47.6331) knots 0 0 0 1 2 2 2
  spline S192 degree 2 poles (45.6476, -47.6331) (45.7242, -47.6331) (45.971, -47.5991) (46.0447, -47.565) knots 0 0 0 1 2 2 2
  spline S193 degree 2 poles (46.0447, -47.565) (46.1355, -47.5253) (46.2631, -47.3807) (46.2631, -47.2644) knots 0 0 0 1 2 2 2
  spline S194 degree 2 poles (46.2631, -47.2644) (46.2631, -47.1311) (46.0561, -46.9666) (45.9143, -46.9297) knots 0 0 0 1 2 2 2
  spline S195 degree 2 poles (45.9143, -46.9297) (45.7356, -46.8815) (45.33, -46.7992) (45.1513, -46.7368) knots 0 0 0 1 2 2 2
  spline S196 degree 2 poles (45.1513, -46.7368) (44.7457, -46.595) (44.394, -46.11) (44.394, -45.747) knots 0 0 0 1 2 2 2
  spline S197 degree 2 poles (44.394, -45.747) (44.394, -45.2563) (45.225, -44.6465) (45.849, -44.6465) knots 0 0 0 1 2 2 2
  spline S198 degree 2 poles (45.849, -44.6465) (46.161, -44.6465) (46.7793, -44.7741) (47.0232, -44.8819) knots 0 0 0 1 2 2 2
  line L172 (47.0232, -44.8819) -> (47.0232, -45.6817)
  line L173 (47.0232, -45.6817) -> (46.9467, -45.6817)
  spline S199 degree 2 poles (46.9467, -45.6817) (46.751, -45.5144) (46.1894, -45.2847) (45.8944, -45.2847) knots 0 0 0 1 2 2 2
  spline S200 degree 2 poles (45.8944, -45.2847) (45.7781, -45.2847) (45.5966, -45.3187) (45.4945, -45.3641) knots 0 0 0 1 2 2 2
  spline S201 degree 2 poles (45.4945, -45.3641) (45.4122, -45.4009) (45.2931, -45.5484) (45.2931, -45.6392) knots 0 0 0 1 2 2 2
  spline S202 degree 2 poles (45.2931, -45.6392) (45.2931, -45.7753) (45.4831, -45.9313) (45.7554, -45.9937) knots 0 0 0 1 2 2 2
  spline S203 degree 2 poles (45.7554, -45.9937) (45.9313, -46.0334) (46.2574, -46.11) (46.4446, -46.1753) knots 0 0 0 1 2 2 2
  spline S204 degree 2 poles (46.4446, -46.1753) (46.8077, -46.3086) (47.1622, -46.751) (47.1622, -47.1141) knots 0 0 0 1 2 2 2
  spline S205 degree 2 poles (47.1622, -47.1141) (47.1622, -47.6359) (46.3425, -48.2713) (45.6448, -48.2713) knots 0 0 0 1 2 2 2
  line L174 (48.2854, -48.2089) -> (48.2854, -45.3754)
  line L175 (48.2854, -45.3754) -> (47.2501, -45.3754)
  line L176 (47.2501, -45.3754) -> (47.2501, -44.7089)
  line L177 (47.2501, -44.7089) -> (50.1999, -44.7089)
  line L178 (50.1999, -44.7089) -> (50.1999, -45.3754)
  line L179 (50.1999, -45.3754) -> (49.1647, -45.3754)
  line L180 (49.1647, -45.3754) -> (49.1647, -48.2089)
  line L181 (49.1647, -48.2089) -> (48.2854, -48.2089)
  line L182 (50.1829, -48.2089) -> (51.3656, -44.7089)
  line L183 (51.3656, -44.7089) -> (52.3243, -44.7089)
  line L184 (52.3243, -44.7089) -> (53.507, -48.2089)
  line L185 (53.507, -48.2089) -> (52.6023, -48.2089)
  line L186 (52.6023, -48.2089) -> (52.3839, -47.4941)
  line L187 (52.3839, -47.4941) -> (51.2834, -47.4941)
  line L188 (51.2834, -47.4941) -> (51.0621, -48.2089)
  line L189 (51.0621, -48.2089) -> (50.1829, -48.2089)
  line L190 (52.191, -46.8588) -> (51.8336, -45.7016)
  line L191 (51.8336, -45.7016) -> (51.4734, -46.8588)
  line L192 (51.4734, -46.8588) -> (52.191, -46.8588)
  point P0 (0, 0)
  constraints: 4 other